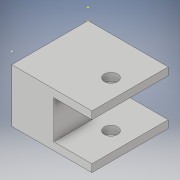
# Autodesk Inventor part: Encaixe Bandeja-Motor
Saved by Autodesk Inventor 2017 (Build 210142000, 142)
## iProperties
Created: 2016-07-16
Part Number: Encaixe Bandeja-Motor
Material: Generic
Document SubType Name: Modeling
Designer: mateu
Density: 1 g/cm^3
Appearance: Default
Author: mateu
Autodesk Inventor part; units mm, degrees
ref_plane "YZ Plane" through (0, 0, 0) normal (1, 0, 0) x (0, 1, 0)
ref_plane "XZ Plane" through (0, 0, 0) normal (0, 1, 0) x (-1, 0, 0)
ref_plane "XY Plane" through (0, 0, 0) normal (0, 0, 1) x (1, 0, 0)
sketch "Sketch1" plane through (0, 0, 0) normal (0, 0, 1) x (1, 0, 0)
  line L0 (0, 0) -> (0, -20)
  line L1 (0, -20) -> (21, -20)
  line L2 (21, -20) -> (21, -15)
  line L3 (21, -15) -> (11, -15)
  line L4 (11, -15) -> (11, -5)
  line L5 (11, -5) -> (21, -5)
  line L6 (21, -5) -> (21, 0)
  line L7 (21, 0) -> (0, 0)
  dimension "d0" = 20
  dimension "d1" = 21
  dimension "d2" = 5
  dimension "d3" = 10
  dimension "d4" = 10
  dimension "d5" = 90
  constraints: 16 end point, 5 perpendicular, 2 point on line, 1 horizontal, 1 vertical
  measures "d0" distance of L0.start L0.end
  measures "d1" distance of L0.end L1.end
  measures "d2" distance of L1.end L2.end
  measures "d3" distance of L2.end L3.end
  measures "d4" distance of L3.end L4.end
  measures "d5" angle of L3 L4
extrude "Extrusion1" add sketch "Sketch1" along normal blind 20
sketch "Sketch2" plane through (0, 0, 20) normal (0, 0, 1) x (1, 0, 0)
  point P0 (0, 0)
sketch "Sketch3" plane through (0, -20, 0) normal (-1, 0, 0) x (0, 0, 1)
  point P0 (0, 20)
sketch "Sketch4" plane through (0, -20, 0) normal (-1, 0, 0) x (0, 0, 1)
  line L0 (20, 20) -> (20, 0) projected
  line L1 (0, 20) -> (20, 20)
  line L2 (20, 20) -> (20, 0)
  line L3 (20, 0) -> (0, 0)
  line L4 (0, 0) -> (0, 20)
  circle A0 centre (10, 10) radius 2.75
  dimension "d8" = 5.5
  dimension "d9" = 10
  dimension "d10" = 10
  constraints: 8 end point, 2 parallel, 1 centre point, 1 horizontal, 1 perpendicular
  measures "d8" diameter of A0
  measures "d9" distance from line of L1 A0.centre
  measures "d10" distance from line of L4 A0.centre
extrude "Extrusion2" cut sketch "Sketch4" against normal blind 11 contours A0
sketch "Sketch5" plane through (0, 0, 0) normal (0, 1, 0) x (1, 0, 0)
  point P0 (0, 0)
sketch "Sketch6" plane through (0, 0, 0) normal (0, 1, 0) x (1, 0, 0)
  line L0 (21, 0) -> (21, -20) projected
  line L1 (0, 0) -> (21, 0)
  line L2 (21, 0) -> (21, -20)
  line L3 (21, -20) -> (0, -20)
  line L4 (0, -20) -> (0, 0)
  constraints: 8 end point, 2 parallel, 1 horizontal, 1 perpendicular
extrude "Extrusion3" cut sketch "Sketch6" against normal blind 3
sketch "Sketch7" plane through (0, -20, 0) normal (0, -1, 0) x (1, 0, 0)
  line L0 (0, 0) -> (21, 0) projected
  line L1 (0, 20) -> (21, 20) projected
  line L2 (0, 0) -> (21, 0)
  line L3 (21, 0) -> (21, 20)
  line L4 (21, 20) -> (0, 20)
  line L5 (0, 20) -> (0, 0)
  constraints: 8 end point, 2 parallel, 1 horizontal, 1 perpendicular
extrude "Extrusion4" cut sketch "Sketch7" against normal blind 3
sketch "Sketch8" plane through (0, -3, 0) normal (0, 1, 0) x (1, 0, 0)
  point P0 (0, 0)
sketch "Sketch9" plane through (0, -3, 0) normal (0, 1, 0) x (1, 0, 0)
  line L0 (0, -20) -> (21, -20) projected
  line L1 (0, 0) -> (21, 0)
  line L2 (21, 0) -> (21, -20)
  line L3 (21, -20) -> (0, -20)
  line L4 (0, -20) -> (0, 0)
  line L5 (0, 0) -> (21, 0) projected
  line L6 (0, 0) -> (11, 0)
  line L7 (11, 0) -> (11, -20)
  circle A0 centre (16, -10) radius 1.75
  dimension "d17" = 11
  dimension "d18" = 3.5
  dimension "d19" = 5
  dimension "d20" = 10
  constraints: 12 end point, 2 parallel, 2 perpendicular, 2 point on line, 1 centre point, 1 horizontal
  measures "d17" distance of L1.start L6.end
  measures "d18" diameter of A0
  measures "d19" distance from line of L2 A0.centre
  measures "d20" distance from line of L0 A0.centre
extrude "Extrusion5" cut sketch "Sketch9" against normal blind 3.5 contours A0
sketch "Sketch10" plane through (0, -17, 0) normal (0, -1, 0) x (1, 0, 0)
  line L0 (11, 20) -> (21, 20) projected
  line L1 (0, 0) -> (21, 0)
  line L2 (21, 0) -> (21, 20)
  line L3 (21, 20) -> (0, 20)
  line L4 (0, 20) -> (0, 0)
  line L5 (11, 0) -> (11, 20) projected
  line L6 (11, 20) -> (11, 0)
  circle A0 centre (16, 10) radius 1.75
  dimension "d23" = 3.5
  dimension "d24" = 5
  dimension "d25" = 10
  constraints: 10 end point, 3 equal length, 1 centre point, 1 horizontal, 1 perpendicular
  measures "d23" diameter of A0
  measures "d24" distance from line of L2 A0.centre
  measures "d25" distance from line of L3 A0.centre
extrude "Extrusion6" cut sketch "Sketch10" against normal blind 3.5 contours A0
body "Solid1"
